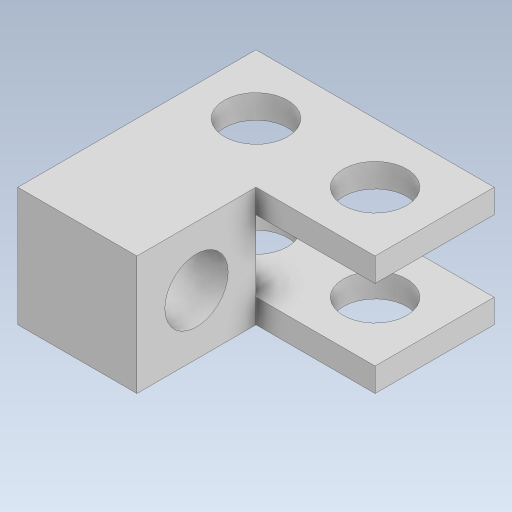
# Autodesk Inventor part: Locker
Saved by Autodesk Inventor 2023 (Build 270158000, 158)
## iProperties
Created: 2022-09-14
Part Number: Locker
Material: Generic
Document SubType Name: Modeling
Designer: Dave
Density: 1 g/cm^3
Appearance: Default
Author: Dave
Autodesk Inventor part; units mm, degrees
ref_plane "YZ Plane" through (0, 0, 0) normal (1, 0, 0) x (0, 1, 0)
ref_plane "XZ Plane" through (0, 0, 0) normal (0, 1, 0) x (-1, 0, 0)
ref_plane "XY Plane" through (0, 0, 0) normal (0, 0, 1) x (1, 0, 0)
sketch "Sketch1" plane through (0, 0, 0) normal (0, 1, 0) x (-1, 0, 0)
  line L0 (0, 0) -> (0, -12.7)
  line L1 (0, -12.7) -> (25.4, -12.7)
  line L2 (25.4, -12.7) -> (25.4, 12.7)
  line L3 (25.4, 12.7) -> (12.7, 12.7)
  line L4 (12.7, 12.7) -> (12.7, 0)
  line L5 (12.7, 0) -> (0, 0)
  dimension "d0" = 12.7
  dimension "d1" = 25.4
  dimension "d2" = 25.4
  dimension "d3" = 12.7
  constraints: 12 end point, 5 perpendicular, 1 vertical
  measures "d0" distance of L0.start L0.end
  measures "d1" distance of L0.end L1.end
  measures "d2" distance of L1.end L2.end
  measures "d3" distance of L4.end L0.start
extrude "Extrusion1" add sketch "Sketch1" along normal blind 12.7
sketch "Sketch2" plane through (-25.4, 0, -12.7) normal (-1, 0, 0) x (0, 0, 1)
  line L0 (25.4, 0) -> (25.4, 12.7) projected
  point P0 (12.7, 0)
  point P1 (19.05, 6.35)
  point P2 (25.4, 6.35)
  dimension "d6" = 6.35
  constraints: 1 horizontal alignment, 1 midpoint
  measures "d6" distance from line of point (19.05, 6.35) L0
sketch "Sketch3" plane through (0, 0, -12.7) normal (0, 0, -1) x (-1, 0, 0)
  line L0 (0, 0) -> (0, 12.7) projected
  line L1 (12.7, 0) -> (12.7, 12.7) projected
  line L2 (0, 10.16) -> (12.7, 10.16)
  line L3 (12.7, 10.16) -> (12.7, 2.54)
  line L4 (12.7, 2.54) -> (0, 2.54)
  line L5 (0, 2.54) -> (0, 10.16)
  line L6 (25.4, 0) -> (25.4, 12.7) projected
  line L7 (12.7, 2.54) -> (25.4, 2.54)
  line L8 (25.4, 2.54) -> (25.4, 10.16)
  line L9 (25.4, 10.16) -> (12.7, 10.16)
  line L10 (12.7, 10.16) -> (12.7, 2.54)
  point P0 (12.7, 6.35)
  point P1 (0, 2.54)
  dimension "d15" = 7.62
  constraints: 16 end point, 4 parallel, 3 point on line, 2 horizontal, 2 midpoint, 2 perpendicular
  measures "d15" distance of L4.end L2.start
extrude "Extrusion2" cut sketch "Sketch3" against normal blind 12.7
sketch "Sketch4" plane through (0, 12.7, 0) normal (0, 1, 0) x (1, 0, 0)
  line L0 (0, 0) -> (0, 12.7) projected
  line L1 (-12.7, 0) -> (0, 0) projected
  line L2 (-12.7, -12.7) -> (-12.7, 0) projected
  line L3 (-12.7, 0) -> (-12.7, 12.7)
  point P0 (-6.35, 6.35)
  point P1 (0, 6.35)
  point P2 (-6.35, 0)
  point P3 (-19.05, 6.35)
  constraints: 2 end point, 2 midpoint, 1 horizontal alignment, 1 symmetric about line, 1 vertical, 1 vertical alignment
hole "Hole2" at (-6.35, 12.7, -6.35) at (-19.05, 12.7, -6.35) direction (0, -1, 0) diameter 6.7564 depth 12.7 tip angle 118 clearance for "Flat Head Machine Screw (82)" size "1/4" standard "Ansi Unified Screw Threads"
hole "Hole3" at (-25.4, 6.35, 6.35) direction (1, 0, 0) diameter 6.7564 depth 12.7 tip angle 118 clearance for "Flat Head Machine Screw (82)" size "1/4" standard "Ansi Unified Screw Threads"
ref_plane "Work Plane1" through (-6.35, 12.7, 0) normal (1, 0, 0) x (0, 0, -1)
body "Solid1"
